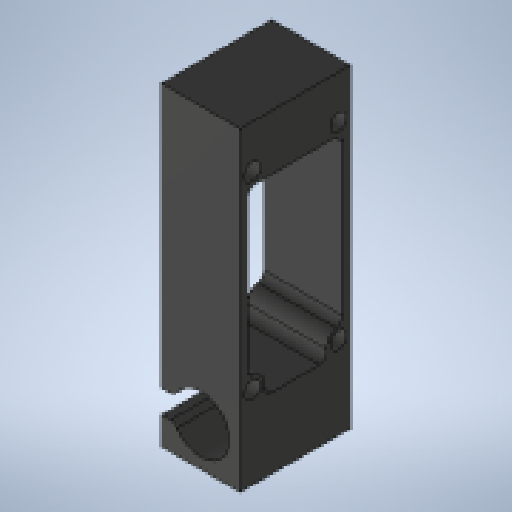
# Autodesk Inventor part: Pod
Saved by Autodesk Inventor 2023.4 (Build 274418000, 418)
## iProperties
Created: 2024-05-08
Part Number: Pod
Material: Rubber, Silicone
Document SubType Name: Modeling
Designer: Nathan Cai
Density: 1.25 g/cm^3
Appearance: Rubber - Black
Author: Nathan Cai
Autodesk Inventor part; units mm, degrees
ref_plane "YZ Plane" through (0, 0, 0) normal (1, 0, 0) x (0, 1, 0)
ref_plane "XZ Plane" through (0, 0, 0) normal (0, 1, 0) x (-1, 0, 0)
ref_plane "XY Plane" through (0, 0, 0) normal (0, 0, 1) x (1, 0, 0)
sketch "Sketch1" plane through (0, 0, 0) normal (1, 0, 0) x (0, 1, 0)
  line L0 (0, 0) -> (127, 0)
  line L1 (127, 0) -> (127, -44.45)
  line L2 (127, -44.45) -> (0, -44.45)
  line L3 (0, -44.45) -> (0, 0)
  line L4 (15.875, -44.45) -> (15.875, 0) construction
  line L5 (28.575, -44.45) -> (28.575, 0)
  line L6 (28.575, -44.45) -> (127, 0) construction
  line L7 (127, -44.45) -> (28.575, 0) construction
  arc A0 (28.575, -4.7625) -> (33.3375, 0) centre (33.3375, -4.7625) ccw
  circle A1 centre (33.3375, -4.7625) radius 3.3655
  line L8 (28.575, -22.225) -> (127, -22.225) construction
  line L9 (37.8276, -41.275) -> (98.425, -41.275)
  line L10 (98.425, -41.275) -> (98.425, -3.175)
  line L11 (98.425, -3.175) -> (37.8276, -3.175)
  arc A2 (33.3375, -44.45) -> (28.575, -39.6875) centre (33.3375, -39.6875) ccw
  circle A3 centre (33.3375, -39.6875) radius 3.3655
  circle A4 centre (103.1875, -39.6875) radius 4.7625 construction
  circle A5 centre (103.1875, -39.6875) radius 3.3655
  circle A6 centre (103.1875, -4.7625) radius 4.7625 construction
  circle A7 centre (103.1875, -4.7625) radius 3.3655
  point P0 (77.7875, -22.225)
  dimension "d0" = 127
  dimension "d1" = 44.45
  dimension "d2" = 15.875
  dimension "d4" = 12.7
  dimension "d5" = 9.525
  dimension "d6" = 6.731
  dimension "d7" = 3.175
  dimension "d8" = 3.175
  dimension "d9" = 69.85
  dimension "d10" = 9.525
  dimension "d11" = 6.731
  constraints: 24 end point, 8 centre point, 6 point on circle, 6 point on line, 6 symmetric about line, 4 coincident, 4 perpendicular, 4 tangent, 3 midpoint, 3 parallel, 1 horizontal, 4 other
  measures "d0" distance of L1.end L2.end
  measures "d1" distance of L0.end L1.end
  measures "d2" distance between parallel lines of L3 L4
  measures "d4" distance between parallel lines of L5 L4
  measures "d5" diameter of A0
  measures "d6" diameter of A1
  measures "d7" distance between parallel lines of L2 L9
  measures "d8" distance between parallel lines of L0 L11
  measures "d9" distance between parallel lines of L5 L10
  measures "d10" diameter of A4
  measures "d11" diameter of A5
extrude "Extrusion1" add sketch "Sketch1" against normal blind 31.75 contours L0 L5 L2 L3 | L0 A0 L5 | L0 L1 L2 A2 L9 L10 L11 A0 | L5 A2 L2
fillet "Fillet1" radius 3.175 6 edges at (-15.875, 28.575, -39.6875) (-15.875, 37.8276, -41.275) (-15.875, 98.425, -41.275) (-15.875, 98.425, -3.175) (-15.875, 37.8276, -3.175) (-15.875, 28.575, -4.7625)
sketch "Sketch2" plane through (0, 0, 0) normal (0, 0, 1) x (1, 0, 0)
  line L0 (0, 0) -> (-31.75, 0) construction
  line L1 (-15.875, 0) -> (-15.875, 127) construction
  line L2 (0, 127) -> (-31.75, 127) construction
  circle A0 centre (-15.875, 15.875) radius 11.5
  line L3 (-38.875, 11.1125) -> (-15.875, 11.1125)
  line L4 (-15.875, 11.1125) -> (-15.875, 20.6375)
  line L5 (-15.875, 20.6375) -> (-38.875, 20.6375)
  line L6 (-38.875, 20.6375) -> (-38.875, 11.1125)
  line L7 (-38.875, 11.1125) -> (-15.875, 20.6375) construction
  line L8 (-15.875, 11.1125) -> (-38.875, 20.6375) construction
  line L9 (-15.875, 15.875) -> (-27.375, 15.875) construction
  point P0 (-26.3425, 11.1125)
  point P1 (-26.3425, 20.6375)
  dimension "d15" = 23
  dimension "d16" = 15.875
  dimension "d17" = 9.525
  constraints: 16 end point, 4 midpoint, 3 point on line, 2 horizontal, 2 parallel, 2 point on circle, 1 centre point, 1 perpendicular
  measures "d15" diameter of A0
  measures "d16" distance from line of L0 L9.start
  measures "d17" distance of L4.end L3.end
extrude "Extrusion2" cut sketch "Sketch2" against normal through all
fillet "Fillet2" radius 3.175 2 edges at (-26.3425, 11.1125, -22.225) (-26.3425, 20.6375, -22.225)
equation "\"d8\" = d7"
body "Solid1"
